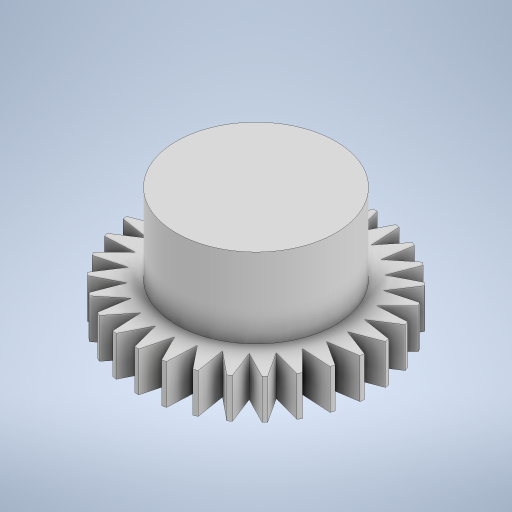
# Autodesk Inventor part: PlanetaryGear
Saved by Autodesk Inventor 2024 (Build 280153000, 153)
## iProperties
Created: 2023-07-07
Part Number: PlanetaryGear
Material: Generic
Document SubType Name: Modeling
Designer: westy
Density: 1 g/cm^3
Appearance: Default
Author: westy
Autodesk Inventor part; units mm, degrees
ref_plane "YZ Plane" through (0, 0, 0) normal (1, 0, 0) x (0, 1, 0)
ref_plane "XZ Plane" through (0, 0, 0) normal (0, 1, 0) x (-1, 0, 0)
ref_plane "XY Plane" through (0, 0, 0) normal (0, 0, 1) x (1, 0, 0)
sketch "Sketch1" plane through (0, 0, 0) normal (0, 1, 0) x (-1, 0, 0)
  circle A0 centre (0, 0) radius 15
  line L0 (14.942, 1.3178) -> (11.506, 0)
  line L1 (11.506, 0) -> (14.942, -1.3178)
  line L2 (14.3415, 4.3956) -> (11.2545, 2.3922)
  line L3 (11.2545, 2.3922) -> (14.8895, 1.8176)
  line L4 (13.1142, 7.2813) -> (10.5112, 4.6799)
  line L5 (10.5112, 4.6799) -> (14.1862, 4.8736)
  line L6 (11.3137, 9.8488) -> (9.3085, 6.763)
  line L7 (9.3085, 6.763) -> (12.8629, 7.7166)
  line L8 (9.0188, 11.9859) -> (7.699, 8.5506)
  line L9 (7.699, 8.5506) -> (10.9775, 10.2223)
  line L10 (6.3297, 13.5991) -> (5.753, 9.9645)
  line L11 (5.753, 9.9645) -> (8.6123, 12.2812)
  line L12 (3.364, 14.6179) -> (3.5555, 10.9428)
  line L13 (3.5555, 10.9428) -> (5.8706, 13.8035)
  line L14 (0.2513, 14.9979) -> (1.2027, 11.4429)
  line L15 (1.2027, 11.4429) -> (2.8725, 14.7224)
  line L16 (-2.8725, 14.7224) -> (-1.2027, 11.4429)
  line L17 (-1.2027, 11.4429) -> (-0.2513, 14.9979)
  line L18 (-5.8706, 13.8035) -> (-3.5555, 10.9428)
  line L19 (-3.5555, 10.9428) -> (-3.364, 14.6179)
  line L20 (-8.6123, 12.2812) -> (-5.753, 9.9645)
  line L21 (-5.753, 9.9645) -> (-6.3297, 13.5991)
  line L22 (-10.9775, 10.2223) -> (-7.699, 8.5506)
  line L23 (-7.699, 8.5506) -> (-9.0188, 11.9859)
  line L24 (-12.8629, 7.7166) -> (-9.3085, 6.763)
  line L25 (-9.3085, 6.763) -> (-11.3137, 9.8488)
  line L26 (-14.1862, 4.8736) -> (-10.5112, 4.6799)
  line L27 (-10.5112, 4.6799) -> (-13.1142, 7.2813)
  line L28 (-14.8895, 1.8176) -> (-11.2545, 2.3922)
  line L29 (-11.2545, 2.3922) -> (-14.3415, 4.3956)
  line L30 (-14.942, -1.3178) -> (-11.506, 0)
  line L31 (-11.506, 0) -> (-14.942, 1.3178)
  line L32 (-14.3415, -4.3956) -> (-11.2545, -2.3922)
  line L33 (-11.2545, -2.3922) -> (-14.8895, -1.8176)
  line L34 (-13.1142, -7.2813) -> (-10.5112, -4.6799)
  line L35 (-10.5112, -4.6799) -> (-14.1862, -4.8736)
  line L36 (-11.3137, -9.8488) -> (-9.3085, -6.763)
  line L37 (-9.3085, -6.763) -> (-12.8629, -7.7166)
  line L38 (-9.0188, -11.9859) -> (-7.699, -8.5506)
  line L39 (-7.699, -8.5506) -> (-10.9775, -10.2223)
  line L40 (-6.3297, -13.5991) -> (-5.753, -9.9645)
  line L41 (-5.753, -9.9645) -> (-8.6123, -12.2812)
  line L42 (-3.364, -14.6179) -> (-3.5555, -10.9428)
  line L43 (-3.5555, -10.9428) -> (-5.8706, -13.8035)
  line L44 (-0.2513, -14.9979) -> (-1.2027, -11.4429)
  line L45 (-1.2027, -11.4429) -> (-2.8725, -14.7224)
  line L46 (2.8725, -14.7224) -> (1.2027, -11.4429)
  line L47 (1.2027, -11.4429) -> (0.2513, -14.9979)
  line L48 (5.8706, -13.8035) -> (3.5555, -10.9428)
  line L49 (3.5555, -10.9428) -> (3.364, -14.6179)
  line L50 (8.6123, -12.2812) -> (5.753, -9.9645)
  line L51 (5.753, -9.9645) -> (6.3297, -13.5991)
  line L52 (10.9775, -10.2223) -> (7.699, -8.5506)
  line L53 (7.699, -8.5506) -> (9.0188, -11.9859)
  line L54 (12.8629, -7.7166) -> (9.3085, -6.763)
  line L55 (9.3085, -6.763) -> (11.3137, -9.8488)
  line L56 (14.1862, -4.8736) -> (10.5112, -4.6799)
  line L57 (10.5112, -4.6799) -> (13.1142, -7.2813)
  line L58 (14.8895, -1.8176) -> (11.2545, -2.3922)
  line L59 (11.2545, -2.3922) -> (14.3415, -4.3956)
  dimension "d0" = 30
  dimension "d3" = 360
  constraints: 120 end point, 1 coincident, 155 other
extrude "Extrusion1" add sketch "Sketch1" along normal blind 5 contours L0 L1 A0 L58 L59 L56 L57 L54 L55 L52 L53 L50 L51 L48 L49 L46 L47 L44 L45 L42 L43 L40 L41 L38 L39 L36 L37 L34 L35 L32 L33 L30 L31 L28 L29 L26 L27 L24 L25 L22 L23 L20 L21 L18 L19 L16 L17 L14 L15 L12 L13 L10 L11 L8 L9 L6 L7 L4 L5 L2 L3
sketch "Sketch2" plane through (0, 0, 0) normal (0, -1, 0) x (1, 0, 0)
  circle A0 centre (0, 0) radius 10.5
  circle A1 centre (0, 0) radius 7.5
  dimension "d7" = 3
  dimension "d8" = 15
  constraints: 2 centre point, 2 coincident
  measures "d7" radial gap between concentric circles of A0 A1
  measures "d8" diameter of A1
extrude "Extrusion2" cut sketch "Sketch2" against normal blind 3
sketch "Sketch3" plane through (0, 5, 0) normal (0, 1, 0) x (1, 0, 0)
  circle A0 centre (0, 0) radius 10
  dimension "d11" = 20
  constraints: 1 centre point, 1 coincident
  measures "d11" diameter of A0
extrude "Extrusion3" add sketch "Sketch3" along normal blind 10
body "Solid1"
